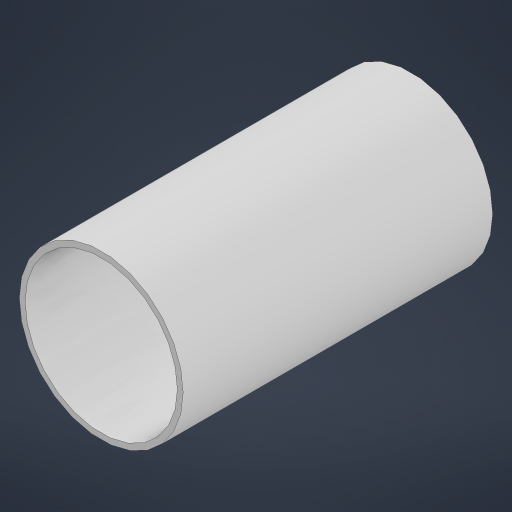
# Autodesk Inventor part: mesh intake part
Saved by Autodesk Inventor 2023.4 (Build 274418000, 418)
## iProperties
Created: 2023-12-04
Part Number: mesh intake part
Material: Generic
Document SubType Name: Modeling
Designer: diego
Density: 1 g/cm^3
Appearance: Default
Author: diego
Autodesk Inventor part; units mm, degrees
ref_plane "YZ Plane" through (0, 0, 0) normal (1, 0, 0) x (0, 1, 0)
ref_plane "XZ Plane" through (0, 0, 0) normal (0, 1, 0) x (-1, 0, 0)
ref_plane "XY Plane" through (0, 0, 0) normal (0, 0, 1) x (1, 0, 0)
sketch "Sketch1" plane through (0, 0, 0) normal (0, 0, 1) x (1, 0, 0)
  circle A0 centre (-11.0418, 22.8376) radius 42.3545
  circle A1 centre (-11.0418, 22.8376) radius 39.37
  point P0 (0, 0)
  dimension "d0" = 84.709
  dimension "d1" = 78.74
  constraints: 2 centre point, 1 coincident
  measures "d0" diameter of A0
  measures "d1" diameter of A1
extrude "Extrusion1" add sketch "Sketch1" along normal blind 160.02
body "Solid1"
